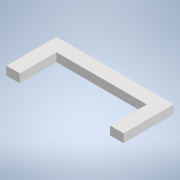
# Autodesk Inventor part: FrameV1
Saved by Autodesk Inventor 2020 (Build 240168000, 168)
## iProperties
Created: 2020-06-07
Part Number: FrameV1
Material: Generic
Document SubType Name: Modeling
Designer: Kitte_x
Density: 1 g/cm^3
Appearance: Default
Author: Kitte_x
Autodesk Inventor part; units mm, degrees
ref_plane "YZ Plane" through (0, 0, 0) normal (1, 0, 0) x (0, 1, 0)
ref_plane "XZ Plane" through (0, 0, 0) normal (0, 1, 0) x (-1, 0, 0)
ref_plane "XY Plane" through (0, 0, 0) normal (0, 0, 1) x (1, 0, 0)
sketch "Sketch1" plane through (0, 0, 0) normal (0, 1, 0) x (-1, 0, 0)
  line L0 (43.65, 37.3) -> (43.65, 0) projected
  line L1 (-50, 0) -> (50, 0) projected
  line L2 (-43.65, 37.3) -> (-43.65, 0) projected
  line L3 (43.65, 37.3) -> (-43.65, 37.3)
  line L4 (12.5, 13.65) -> (-12.5, 13.65)
  line L5 (-12.5, 13.65) -> (-12.5, 23.65)
  line L6 (-12.5, 23.65) -> (12.5, 23.65)
  line L7 (12.5, 23.65) -> (12.5, 13.65)
  circle A0 centre (17.5, 18.65) radius 2.5
  circle A1 centre (-17.5, 18.65) radius 2.5
  point P0 (0, 0)
  point P1 (-33.65, 37.3)
  point P2 (-12.5, 18.65)
  point P3 (12.5, 18.65)
  point P4 (-43.65, 18.65)
  point P5 (0, 0)
  point P6 (0, 13.65)
  dimension "d5" = 25
  dimension "d6" = 10
  dimension "d7" = 5
  dimension "d8" = 5
  dimension "d9" = 5
  dimension "d10" = 5
  constraints: 10 end point, 5 midpoint, 3 horizontal alignment, 2 centre point, 2 horizontal, 2 parallel, 1 perpendicular, 1 vertical alignment
  measures "d5" distance of L5.end L6.end
  measures "d6" distance of L4.end L5.end
  measures "d7" diameter of A0
  measures "d8" diameter of A1
  measures "d9" distance of point (-12.5, 18.65) A1.centre
  measures "d10" distance from line of L7 A0.centre
extrude "Extrusion2" add sketch "Sketch1" along normal blind 6.35
body "Solid2"
